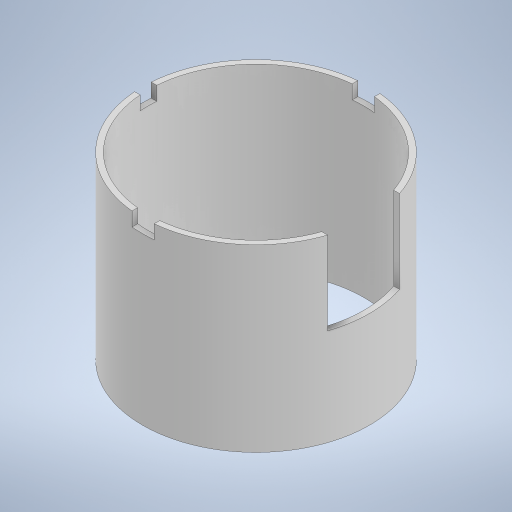
# Autodesk Inventor part: case
Saved by Autodesk Inventor 2024 (Build 280153000, 153)
## iProperties
Created: 2024-05-21
Part Number: case
Material: Generic
Document SubType Name: Modeling
Designer: ryana
Density: 1 g/cm^3
Appearance: Default
Author: ryana
Autodesk Inventor part; units mm, degrees
ref_plane "YZ Plane" through (0, 0, 0) normal (1, 0, 0) x (0, 1, 0)
ref_plane "XZ Plane" through (0, 0, 0) normal (0, 1, 0) x (-1, 0, 0)
ref_plane "XY Plane" through (0, 0, 0) normal (0, 0, 1) x (1, 0, 0)
sketch "Sketch1" plane through (0, 0, 0) normal (0, 1, 0) x (-1, 0, 0)
  circle A0 centre (0, 0) radius 41
  circle A1 centre (0, 0) radius 39
  dimension "d0" = 82
  dimension "d1" = 78
  constraints: 2 centre point, 2 coincident
  measures "d0" diameter of A0
  measures "d1" diameter of A1
extrude "Extrusion1" add sketch "Sketch1" along normal blind 65
sketch "Sketch2" plane through (0, 65, 0) normal (0, 1, 0) x (1, 0, 0)
  line L0 (-4, -41) -> (4, -41)
  line L1 (4, -41) -> (4, 41)
  line L2 (4, 41) -> (-4, 41)
  line L3 (-4, 41) -> (-4, -41)
  line L4 (-4, -41) -> (4, 41) construction
  line L5 (4, -41) -> (-4, 41) construction
  point P0 (0, 0)
  dimension "d4" = 8
  dimension "d5" = 82
  constraints: 12 end point, 2 midpoint, 2 parallel, 1 horizontal, 1 perpendicular
  measures "d4" distance of L2.end L1.end
  measures "d5" distance of L1.end L0.end
extrude "Extrusion2" cut sketch "Sketch2" against normal blind 5
sketch "Sketch3" plane through (0, 65, 0) normal (0, 1, 0) x (1, 0, 0)
  line L0 (-41, 3) -> (-41, -3)
  line L1 (-41, -3) -> (41, -3)
  line L2 (41, -3) -> (41, 3)
  line L3 (41, 3) -> (-41, 3)
  line L4 (-41, 3) -> (41, -3) construction
  line L5 (-41, -3) -> (41, 3) construction
  line L6 (-41, 3) -> (-35, 3) construction
  point P0 (0, 0)
  dimension "d8" = 6
  dimension "d9" = 90
  dimension "d10" = 82
  constraints: 14 end point, 2 midpoint, 2 parallel, 2 perpendicular, 1 horizontal, 1 vertical
  measures "d8" distance of L0.start L0.end
  measures "d9" angle of L0 L6
  measures "d10" distance of L1.end L0.end
extrude "Extrusion3" cut sketch "Sketch3" against normal blind 5
sketch "Sketch4" plane through (0, 65, 0) normal (0, 1, 0) x (1, 0, 0)
  line L0 (0, 0) -> (0, 13)
  line L1 (0, 13) -> (0, -13)
  line L2 (0, -13) -> (82, -13)
  line L3 (82, -13) -> (82, 13)
  line L4 (82, 13) -> (0, 13)
  dimension "d13" = 13
  dimension "d14" = 26
  dimension "d15" = 82
  constraints: 10 end point, 2 parallel, 1 perpendicular, 1 point on line, 1 vertical
  measures "d13" distance of L0.start L0.end
  measures "d14" distance of L0.end L1.end
  measures "d15" distance of L2.end L1.end
extrude "Extrusion4" cut sketch "Sketch4" against normal blind 30
sketch "Sketch5" plane through (0, 0, 0) normal (1, 0, 0) x (0, 1, 0)
  circle A0 centre (0, 0) radius 4
  dimension "d18" = 8
  constraints: 1 centre point, 1 coincident
  measures "d18" diameter of A0
extrude "Extrusion5" cut sketch "Sketch5" against normal blind 82
body "Solid1"
